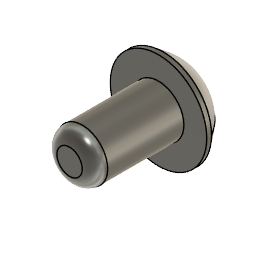
Assembled Parallel Gripper (Autodesk Fusion 360 archive; units mm, degrees)
design "P.Gripper_Pin"
part number: 2026-07-30-16-02-04-406
Autodesk Fusion 360 part; units mm, degrees
sketch "Sketch2" plane through (0, 0, 0) normal (0, 0, 1) x (1, 0, 0)
  line L0 (0, 20) -> (3.8, 20)
  line L1 (3.8, 20) -> (3.8, 20.38)
  spline S0 degree 5 poles (3.8, 20.38) (3.7593, 20.4429) (3.678, 20.5664) (3.5568, 20.7451) (3.3966, 20.9696) (3.1989, 21.2259) (3.0039, 21.4555) (2.812, 21.6558) (2.6234, 21.8246) (2.438, 21.9621) (2.2557, 22.0702) (2.1121, 22.1349) (2.0056, 22.1719) (1.9351, 22.1915) (1.9, 22.2) knots 0 0 0 0 0 0 0.1 0.2 0.3 0.4 0.5 0.6 0.7 0.8 0.9 1 1 1 1 1 1
  line L2 (0, 20) -> (0, 22.2)
  line L3 (0, 22.2) -> (1.9, 22.2)
  point P0 (2.7411, 21.7155)
  dimension "d4" = 3.8
  dimension "d5" = 0.38
  dimension "d6" = 2.2
  dimension "d7" = 1.9
  constraint horizontal L0
  constraint perpendicular L0 L1
  constraint perpendicular L0 L2
  constraint perpendicular L2 L3
  measures "d4" distance of L0.start L0.end
  measures "d5" distance of L0.end L1.end
  measures "d6" distance of L0.start L2.end
  measures "d7" distance of L2.end S0.end
revolve "Revolve1" add sketch "Sketch2" angle 360 about axis through (0, 20, 0) along (0, 1, 0)
sketch "Sketch3" plane through (0, 22.2, 0) normal (0, 1, 0) x (-1, 0, 0)
  circle A0 centre (0, 0) radius 1.9
  line L0 (0.7217, -1.25) -> (1.4434, 0)
  line L1 (1.4434, 0) -> (0.7217, 1.25)
  line L2 (0.7217, 1.25) -> (-0.7217, 1.25)
  line L3 (-0.7217, 1.25) -> (-1.4434, 0)
  line L4 (-1.4434, 0) -> (-0.7217, -1.25)
  line L5 (-0.7217, -1.25) -> (0.7217, -1.25)
  dimension "d9" = 2.5
  constraint coincident A0.centre origin
  measures "d9" distance of L0.start L1.end
extrude "Extrude2" cut sketch "Sketch3" against normal blind 2 contours L0 L1 L2 L3 L4 L5
sketch "Sketch4" plane through (0, 20, 0) normal (0, -1, 0) x (1, 0, 0)
  circle A0 centre (0, 0) radius 3.8
  circle A1 centre (0, 0) radius 2
  dimension "d14" = 4
  constraint coincident A0.centre A1.centre
  measures "d14" diameter of A1
extrude "Extrude3" add sketch "Sketch4" along normal blind 7 contours A1
fillet "Fillet2" radius 1 1 edges at (-1.8647, 13, -0.7232)

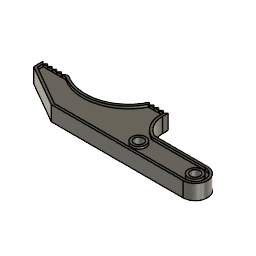
design "P.Gripper_gripper"
part number: 2026-07-22-21-10-46-323
Autodesk Fusion 360 part; units mm, degrees
sketch "Sketch1" plane through (0, 0, 0) normal (0, 0, 1) x (1, 0, 0)
  line L0 (35, 0) -> (-35, 0)
  line L1 (-35, 0) -> (-57.0836, 12.75)
  line L2 (-35, 0) -> (-60.5, 0) construction
  line L3 (-57.0836, 12.75) -> (-57.0836, 17.75)
  line L4 (-57.0836, 17.75) -> (-43.4836, 17.75)
  line L5 (-10, 27.12) -> (0.01, 27.12)
  arc A0 (-43.4836, 17.75) -> (-10, 27.12) centre (-30.7999, 36.9365) ccw
  line L6 (35, 0) -> (35, 13)
  arc A1 (35, 0) -> (35, 13) centre (35, 6.5) ccw
  line L7 (35, 13) -> (6.8247, 13)
  line L8 (0.01, 27.12) -> (0.01, 24.12)
  arc A2 (0.01, 24.12) -> (6.8247, 13) centre (12.49, 24.12) ccw
  dimension "d1" = 70
  dimension "d2" = 30
  dimension "d3" = 25.5
  dimension "d4" = 5
  dimension "d5" = 13.6
  dimension "d6" = 10.01
  dimension "d7" = 27.12
  dimension "d8" = 23
  dimension "d9" = 13
  dimension "d10" = 3
  constraint midpoint L0 origin
  constraint horizontal L0
  constraint horizontal L2
  constraint vertical L3
  constraint perpendicular L3 L4
  constraint horizontal L5
  constraint perpendicular L0 L6
  constraint midpoint L6 A1.centre
  constraint tangent A1 L7
  constraint perpendicular L5 L8
  constraint tangent L8 A2
  measures "d1" distance of L0.start L0.end
  measures "d2" angle of L1 L2
  measures "d3" distance of L0.end L1.end
  measures "d4" distance of L1.end L3.end
  measures "d5" distance of L3.end L4.end
  measures "d6" distance of L5.start L5.end
  measures "d7" distance of L0 L5
  measures "d8" radius of A0
  measures "d9" distance of L0.start L6.end
  measures "d10" distance of L5.end L8.end
extrude "Extrude1" add sketch "Sketch1" along normal mid plane 8
fillet "Fillet1" radius 2 1 edges at (6.8247, 13, 0)
sketch "Sketch2" plane through (0, 0, 4) normal (0, 0, 1) x (-1, 0, 0)
  arc A0 (-35, 0) -> (-35, -13) centre (-35, -6.5) ccw
  line L0 (-35, -13) -> (-7.3271, -13)
  arc A1 (-6.3418, -13.2595) -> (-7.3271, -13) centre (-7.3271, -15) ccw
  arc A2 (-0.01, -24.12) -> (-6.3418, -13.2595) centre (-12.49, -24.12) ccw
  line L1 (-0.01, -24.12) -> (-0.01, -27.12)
  line L2 (-0.01, -27.12) -> (10, -27.12)
  arc A3 (43.4836, -17.75) -> (10, -27.12) centre (30.7999, -36.9365) ccw
  line L3 (43.4836, -17.75) -> (57.0836, -17.75)
  line L4 (57.0836, -17.75) -> (57.0836, -12.75)
  line L5 (57.0836, -12.75) -> (35, 0)
  line L6 (35, 0) -> (-35, 0)
  circle A4 centre (-35, -6.5) radius 2.5
  line L7 (-35, -6.5) -> (-5, -6.5)
  circle A5 centre (-5, -6.5) radius 2.5
  dimension "d15" = 5
  dimension "d16" = 30
  dimension "d17" = 5
  constraint concentric A0 A4
  constraint coincident A0.centre A4.centre
  constraint parallel L0 L7
  constraint coincident L7.end A5.centre
  measures "d15" diameter of A4
  measures "d16" distance of A0.centre L7.end
  measures "d17" diameter of A5
extrude "Extrude2" cut sketch "Sketch2" against normal blind 16 contours A4 | A5
sketch "Sketch3" plane through (0, 0, 4) normal (0, 0, 1) x (-1, 0, 0)
  circle A0 centre (-5, -6.5) radius 2.5
  circle A1 centre (-35, -6.5) radius 2.5
  arc A2 (-35, 0) -> (-35, -13) centre (-35, -6.5) ccw
  line L0 (-35, -13) -> (-7.3271, -13)
  arc A3 (-6.3418, -13.2595) -> (-7.3271, -13) centre (-7.3271, -15) ccw
  arc A4 (-0.01, -24.12) -> (-6.3418, -13.2595) centre (-12.49, -24.12) ccw
  line L1 (-0.01, -24.12) -> (-0.01, -27.12)
  line L2 (-0.01, -27.12) -> (10, -27.12)
  arc A5 (43.4836, -17.75) -> (10, -27.12) centre (30.7999, -36.9365) ccw
  line L3 (43.4836, -17.75) -> (57.0836, -17.75)
  line L4 (57.0836, -17.75) -> (57.0836, -12.75)
  line L5 (57.0836, -12.75) -> (35, 0)
  line L6 (35, 0) -> (-35, 0)
  arc A6 (43.8541, -16.5) -> (9.2223, -25.87) centre (30.7999, -36.9365) ccw
  line L7 (1.24, -25.87) -> (9.2223, -25.87)
  line L8 (1.24, -24.12) -> (1.24, -25.87)
  arc A7 (1.24, -24.12) -> (-5.726, -12.1718) centre (-12.49, -24.12) ccw
  arc A8 (-5.726, -12.1718) -> (-7.3271, -11.75) centre (-7.3271, -15) ccw
  line L9 (-35, -11.75) -> (-7.3271, -11.75)
  arc A9 (-35, -1.25) -> (-35, -11.75) centre (-35, -6.5) ccw
  line L10 (34.6651, -1.25) -> (-35, -1.25)
  line L11 (55.8336, -13.4717) -> (34.6651, -1.25)
  line L12 (55.8336, -16.5) -> (55.8336, -13.4717)
  line L13 (43.8541, -16.5) -> (55.8336, -16.5)
  dimension "d21" = -1.25
extrude "Extrude3" cut sketch "Sketch3" against normal blind 1.25 contours A6 L7 L8 A7 A8 L9 A9 L10 L11 L12 L13
sketch "Sketch4" plane through (0, 0, 2.75) normal (0, 0, 1) x (-1, 0, 0)
  circle A0 centre (-35, -6.5) radius 2.5
  circle A1 centre (-5, -6.5) radius 2.5
  line L0 (1.24, -24.12) -> (1.24, -25.87)
  line L1 (1.24, -25.87) -> (9.2223, -25.87)
  arc A2 (43.8541, -16.5) -> (9.2223, -25.87) centre (30.7999, -36.9365) ccw
  line L2 (43.8541, -16.5) -> (55.8336, -16.5)
  line L3 (55.8336, -16.5) -> (55.8336, -13.4717)
  line L4 (55.8336, -13.4717) -> (34.6651, -1.25)
  line L5 (34.6651, -1.25) -> (-35, -1.25)
  arc A3 (-35, -1.25) -> (-35, -11.75) centre (-35, -6.5) ccw
  line L6 (-35, -11.75) -> (-7.3271, -11.75)
  arc A4 (-5.726, -12.1718) -> (-7.3271, -11.75) centre (-7.3271, -15) ccw
  arc A5 (1.24, -24.12) -> (-5.726, -12.1718) centre (-12.49, -24.12) ccw
  circle A6 centre (-5, -6.5) radius 3.75
  circle A7 centre (-35, -6.5) radius 3.75
  dimension "d24" = 1.25
  dimension "d25" = 1.25
extrude "Extrude4" add sketch "Sketch4" along normal blind 1.25 contours A6 | A7
sketch "Sketch5" plane through (0, 0, -4) normal (0, 0, -1) x (1, 0, 0)
  circle A0 centre (5, -6.5) radius 2.5
  circle A1 centre (35, -6.5) radius 2.5
  arc A2 (35, -13) -> (35, 0) centre (35, -6.5) ccw
  line L0 (35, 0) -> (-35, 0)
  line L1 (-35, 0) -> (-57.0836, -12.75)
  line L2 (-57.0836, -12.75) -> (-57.0836, -17.75)
  line L3 (-57.0836, -17.75) -> (-43.4836, -17.75)
  arc A3 (-10, -27.12) -> (-43.4836, -17.75) centre (-30.7999, -36.9365) ccw
  line L4 (-10, -27.12) -> (0.01, -27.12)
  line L5 (0.01, -27.12) -> (0.01, -24.12)
  arc A4 (6.3418, -13.2595) -> (0.01, -24.12) centre (12.49, -24.12) ccw
  arc A5 (7.3271, -13) -> (6.3418, -13.2595) centre (7.3271, -15) ccw
  line L6 (7.3271, -13) -> (35, -13)
  circle A6 centre (5, -6.5) radius 3.75
  circle A7 centre (35, -6.5) radius 3.75
  line L7 (-55.8336, -16.5) -> (-43.8541, -16.5)
  arc A8 (-9.2223, -25.87) -> (-43.8541, -16.5) centre (-30.7999, -36.9365) ccw
  line L8 (-9.2223, -25.87) -> (-1.24, -25.87)
  line L9 (-1.24, -25.87) -> (-1.24, -24.12)
  arc A9 (5.726, -12.1718) -> (-1.24, -24.12) centre (12.49, -24.12) ccw
  arc A10 (7.3271, -11.75) -> (5.726, -12.1718) centre (7.3271, -15) ccw
  line L10 (7.3271, -11.75) -> (35, -11.75)
  arc A11 (35, -11.75) -> (35, -1.25) centre (35, -6.5) ccw
  line L11 (35, -1.25) -> (-34.6651, -1.25)
  line L12 (-34.6651, -1.25) -> (-55.8336, -13.4717)
  line L13 (-55.8336, -13.4717) -> (-55.8336, -16.5)
  dimension "d28" = 1.25
  dimension "d29" = 1.25
  dimension "d30" = 1.25
extrude "Extrude5" cut sketch "Sketch5" against normal blind 1.25 contours L7 A8 L8 L9 A9 A10 L10 A11 L11 L12 L13
sketch "Sketch7" plane through (0, 0, 4) normal (0, 0, 1) x (-1, 0, 0)
  line L0 (9.2223, -25.87) -> (1.24, -25.87)
  line L1 (1.24, -25.87) -> (1.24, -24.12)
  arc A0 (1.24, -24.12) -> (-5.726, -12.1718) centre (-12.49, -24.12) ccw
  arc A1 (-5.726, -12.1718) -> (-7.3271, -11.75) centre (-7.3271, -15) ccw
  line L2 (-7.3271, -11.75) -> (-35, -11.75)
  arc A2 (-35, -1.25) -> (-35, -11.75) centre (-35, -6.5) ccw
  line L3 (-35, -1.25) -> (34.6651, -1.25)
  line L4 (34.6651, -1.25) -> (55.8336, -13.4717)
  line L5 (55.8336, -13.4717) -> (55.8336, -16.5)
  line L6 (55.8336, -16.5) -> (43.8541, -16.5)
  arc A3 (43.8541, -16.5) -> (9.2223, -25.87) centre (30.7999, -36.9365) ccw
  arc A4 (-35, 0) -> (-35, -13) centre (-35, -6.5) ccw
  line L7 (-35, -13) -> (-7.3271, -13)
  arc A5 (-6.3418, -13.2595) -> (-7.3271, -13) centre (-7.3271, -15) ccw
  arc A6 (-0.01, -24.12) -> (-6.3418, -13.2595) centre (-12.49, -24.12) ccw
  line L8 (-0.01, -24.12) -> (-0.01, -27.12)
  line L9 (-0.01, -27.12) -> (10, -27.12)
  arc A7 (43.4836, -17.75) -> (10, -27.12) centre (30.7999, -36.9365) ccw
  line L10 (43.4836, -17.75) -> (57.0836, -17.75)
  line L11 (57.0836, -17.75) -> (57.0836, -12.75)
  line L12 (57.0836, -12.75) -> (35, 0)
  line L13 (35, 0) -> (-35, 0)
  line L14 (42, -16.7) -> (58, -16.7)
  line L15 (57.0836, -17.75) -> (55.8816, -16.5479)
  line L16 (57.0836, -17.75) -> (58.7836, -17.75) construction
  line L17 (55.8816, -16.5479) -> (54.6795, -17.75)
  line L18 (54.6795, -17.75) -> (53.4525, -16.523)
  line L19 (53.4525, -16.523) -> (52.2254, -17.75)
  line L20 (52.2254, -17.75) -> (50.9984, -16.523)
  line L21 (50.9984, -16.523) -> (49.7714, -17.75)
  line L22 (49.7714, -17.75) -> (48.5214, -16.5)
  line L23 (48.5214, -16.5) -> (47.2714, -17.75)
  line L24 (47.2714, -17.75) -> (46.0214, -16.5)
  line L25 (46.0214, -16.5) -> (44.7714, -17.75)
  line L26 (44.7714, -17.75) -> (43.5093, -16.4879)
  point P0 (50, -16.7)
  dimension "d33" = 0.2
  dimension "d34" = 135
  dimension "d35" = 1.7
  dimension "d37" = 90
  constraint midpoint L14 P0
  constraint perpendicular L11 L14
  constraint horizontal L16
  constraint coincident L10.end L11.start
  constraint coincident L10 L17.end
  constraint perpendicular L15 L17
  constraint coincident L10 L19.end
  constraint perpendicular L18 L19
  constraint coincident L10 L21.end
  constraint perpendicular L20 L21
  constraint coincident L6 L22.end
  constraint perpendicular L21 L22
  constraint coincident L10 L23.end
  constraint perpendicular L22 L23
  constraint coincident L6 L24.end
  constraint perpendicular L23 L24
  constraint coincident L10 L25.end
  constraint perpendicular L24 L25
  measures "d33" distance of L6 L14
  measures "d34" angle of L15 L16
  measures "d35" distance of L10.end L15.end
  measures "d37" angle of L25 L26
extrude "Extrude6" cut sketch "Sketch7" against normal blind 16 contours L10 L14 L24 L25 | L10 L14 L22 L23 | L10 L14 L20 L21 | L10 L14 L18 L19 | L10 L14 L15 L17
sketch "Sketch8" plane through (0, 0, 4) normal (0, 0, 1) x (-1, 0, 0)
  line L0 (9.2223, -25.87) -> (1.24, -25.87)
  line L1 (1.24, -25.87) -> (1.24, -24.12)
  arc A0 (1.24, -24.12) -> (-5.726, -12.1718) centre (-12.49, -24.12) ccw
  arc A1 (-5.726, -12.1718) -> (-7.3271, -11.75) centre (-7.3271, -15) ccw
  line L2 (-7.3271, -11.75) -> (-35, -11.75)
  arc A2 (-35, -1.25) -> (-35, -11.75) centre (-35, -6.5) ccw
  line L3 (-35, -1.25) -> (34.6651, -1.25)
  line L4 (34.6651, -1.25) -> (55.8336, -13.4717)
  line L5 (55.8336, -13.4717) -> (55.8336, -16.5)
  line L6 (55.8336, -16.5) -> (43.8541, -16.5)
  arc A3 (43.8541, -16.5) -> (9.2223, -25.87) centre (30.7999, -36.9365) ccw
  line L7 (44.7714, -17.75) -> (45.8214, -16.7)
  line L8 (45.8214, -16.7) -> (46.2214, -16.7)
  line L9 (46.2214, -16.7) -> (47.2714, -17.75)
  line L10 (47.2714, -17.75) -> (48.3214, -16.7)
  line L11 (48.3214, -16.7) -> (48.7214, -16.7)
  line L12 (48.7214, -16.7) -> (49.7714, -17.75)
  line L13 (49.7714, -17.75) -> (50.8214, -16.7)
  line L14 (50.8214, -16.7) -> (51.1754, -16.7)
  line L15 (51.1754, -16.7) -> (52.2254, -17.75)
  line L16 (52.2254, -17.75) -> (53.2754, -16.7)
  line L17 (53.2754, -16.7) -> (53.6295, -16.7)
  line L18 (53.6295, -16.7) -> (54.6795, -17.75)
  line L19 (54.6795, -17.75) -> (55.7295, -16.7)
  line L20 (55.7295, -16.7) -> (56.0336, -16.7)
  line L21 (56.0336, -16.7) -> (57.0836, -17.75)
  line L22 (57.0836, -17.75) -> (57.0836, -12.75)
  line L23 (57.0836, -12.75) -> (35, 0)
  line L24 (35, 0) -> (-35, 0)
  arc A4 (-35, 0) -> (-35, -13) centre (-35, -6.5) ccw
  line L25 (-35, -13) -> (-7.3271, -13)
  arc A5 (-6.3418, -13.2595) -> (-7.3271, -13) centre (-7.3271, -15) ccw
  arc A6 (-0.01, -24.12) -> (-6.3418, -13.2595) centre (-12.49, -24.12) ccw
  line L26 (-0.01, -24.12) -> (-0.01, -27.12)
  line L27 (-0.01, -27.12) -> (10, -27.12)
  arc A7 (43.4836, -17.75) -> (10, -27.12) centre (30.7999, -36.9365) ccw
  line L28 (43.4836, -17.75) -> (44.7714, -17.75)
  line L29 (-1.01, -26.07) -> (11, -26.07)
  line L30 (10, -27.12) -> (8.75, -25.87)
  line L31 (10, -27.12) -> (11.7678, -27.12) construction
  line L32 (8.75, -25.87) -> (7.5, -27.12)
  line L33 (7.5, -27.12) -> (6.25, -25.87)
  line L34 (6.25, -25.87) -> (4.995, -27.125)
  line L35 (4.995, -27.125) -> (3.74, -25.87)
  line L36 (3.74, -25.87) -> (2.49, -27.12)
  line L37 (2.49, -27.12) -> (1.24, -25.87)
  line L38 (1.24, -25.87) -> (-0.01, -27.12)
  point P0 (4.995, -26.07)
  dimension "d40" = 0.2
  dimension "d41" = 135
  constraint midpoint L29 P0
  constraint parallel L27 L29
  constraint horizontal L31
  constraint coincident L27.end A7.end
  constraint coincident L0 L30.end
  constraint coincident L27 L32.end
  constraint perpendicular L30 L32
  constraint perpendicular L32 L33
  constraint perpendicular L33 L34
  constraint coincident L0 L35.end
  constraint perpendicular L34 L35
  constraint coincident L27 L36.end
  constraint perpendicular L35 L36
  constraint coincident L0.end L1.start
  constraint perpendicular L36 L37
  constraint coincident L26.end L27.start
  measures "d40" distance of L0 L29
  measures "d41" angle of L30 L31
extrude "Extrude7" cut sketch "Sketch8" against normal blind 16 contours L27 L29 L30 L32 | L27 L29 L33 L34 | L27 L29 L35 L36 | L27 L29 L37 L38

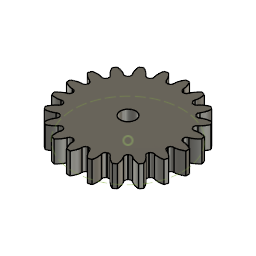
design "Spur Gear 20 teeth"
description: Spur Gear; Module: 1.75; Num Teeth: 20; Pressure Angle: 20.0; Backlash: 0.00 mm
part number: 2026-07-22-22-21-55-407
Autodesk Fusion 360 part; units mm, degrees
sketch "Base Circle" plane through (0, 0, 0) normal (0, 0, 1) x (1, 0, 0)
  circle A0 centre (0, 0) radius 15.4753
  circle A1 centre (0, 0) radius 2.5
extrude "Extrude1" add sketch "Base Circle" along normal blind 7
sketch "Gear Tooth" plane through (0, 0, 0) normal (0, 0, 1) x (1, 0, 0)
  spline S0 degree 5 poles (16.3729, -1.5344) (16.3811, -1.5352) (16.3975, -1.5365) (16.4221, -1.5378) (16.455, -1.5384) (16.4962, -1.5373) (16.5375, -1.535) (16.5788, -1.532) (16.6201, -1.5285) (16.6614, -1.5248) (16.7028, -1.5207) (16.7442, -1.5163) (16.7855, -1.5114) (16.8269, -1.5059) (16.8683, -1.4998) (16.9098, -1.4931) (16.9512, -1.486) (16.9926, -1.4784) (17.034, -1.4706) (17.0754, -1.4623) (17.1168, -1.4538) (17.1582, -1.4449) (17.1996, -1.4356) (17.241, -1.426) (17.2824, -1.416) (17.3238, -1.4057) (17.3651, -1.395) (17.4065, -1.3839) (17.4478, -1.3726) (17.4891, -1.361) (17.5304, -1.349) (17.5717, -1.3368) (17.613, -1.3243) (17.6542, -1.3114) (17.6955, -1.2983) (17.7367, -1.2849) (17.7779, -1.2711) (17.8191, -1.2571) (17.8602, -1.2429) (17.9013, -1.2283) (17.9424, -1.2135) (17.9835, -1.1984) (18.0246, -1.183) (18.0656, -1.1674) (18.1066, -1.1515) (18.1475, -1.1354) (18.1885, -1.119) (18.2294, -1.1023) (18.2703, -1.0854) (18.3111, -1.0682) (18.3519, -1.0508) (18.3927, -1.0331) (18.4334, -1.0152) (18.4742, -0.9971) (18.5148, -0.9787) (18.5555, -0.96) (18.5961, -0.9412) (18.6367, -0.922) (18.6772, -0.9027) (18.7177, -0.8831) (18.7582, -0.8633) (18.7986, -0.8433) (18.839, -0.823) (18.8793, -0.8025) (18.9196, -0.7818) (18.9598, -0.7608) (19.0001, -0.7396) (19.0402, -0.7182) (19.0804, -0.6966) (19.1204, -0.6748) (19.1605, -0.6527) (19.1925, -0.6349) (19.2164, -0.6215) (19.2324, -0.6124) (19.2404, -0.6079) knots 0 0 0 0 0 0 0.01428571 0.02857143 0.04285714 0.05714286 0.07142857 0.08571429 0.1 0.11428571 0.12857143 0.14285714 0.15714286 0.17142857 0.18571429 0.2 0.21428571 0.22857143 0.24285714 0.25714286 0.27142857 0.28571429 0.3 0.31428571 0.32857143 0.34285714 0.35714286 0.37142857 0.38571429 0.4 0.41428571 0.42857143 0.44285714 0.45714286 0.47142857 0.48571429 0.5 0.51428571 0.52857143 0.54285714 0.55714286 0.57142857 0.58571429 0.6 0.61428571 0.62857143 0.64285714 0.65714286 0.67142857 0.68571429 0.7 0.71428571 0.72857143 0.74285714 0.75714286 0.77142857 0.78571429 0.8 0.81428571 0.82857143 0.84285714 0.85714286 0.87142857 0.88571429 0.9 0.91428571 0.92857143 0.94285714 0.95714286 0.97142857 0.98571429 1 1 1 1 1 1
  spline S1 degree 5 poles (16.3729, 1.5344) (16.3811, 1.5352) (16.3975, 1.5365) (16.4221, 1.5378) (16.455, 1.5384) (16.4962, 1.5373) (16.5375, 1.535) (16.5788, 1.532) (16.6201, 1.5285) (16.6614, 1.5248) (16.7028, 1.5207) (16.7442, 1.5163) (16.7855, 1.5114) (16.8269, 1.5059) (16.8683, 1.4998) (16.9098, 1.4931) (16.9512, 1.486) (16.9926, 1.4784) (17.034, 1.4706) (17.0754, 1.4623) (17.1168, 1.4538) (17.1582, 1.4449) (17.1996, 1.4356) (17.241, 1.426) (17.2824, 1.416) (17.3238, 1.4057) (17.3651, 1.395) (17.4065, 1.3839) (17.4478, 1.3726) (17.4891, 1.361) (17.5304, 1.349) (17.5717, 1.3368) (17.613, 1.3243) (17.6542, 1.3114) (17.6955, 1.2983) (17.7367, 1.2849) (17.7779, 1.2711) (17.8191, 1.2571) (17.8602, 1.2429) (17.9013, 1.2283) (17.9424, 1.2135) (17.9835, 1.1984) (18.0246, 1.183) (18.0656, 1.1674) (18.1066, 1.1515) (18.1475, 1.1354) (18.1885, 1.119) (18.2294, 1.1023) (18.2703, 1.0854) (18.3111, 1.0682) (18.3519, 1.0508) (18.3927, 1.0331) (18.4334, 1.0152) (18.4742, 0.9971) (18.5148, 0.9787) (18.5555, 0.96) (18.5961, 0.9412) (18.6367, 0.922) (18.6772, 0.9027) (18.7177, 0.8831) (18.7582, 0.8633) (18.7986, 0.8433) (18.839, 0.823) (18.8793, 0.8025) (18.9196, 0.7818) (18.9598, 0.7608) (19.0001, 0.7396) (19.0402, 0.7182) (19.0804, 0.6966) (19.1204, 0.6748) (19.1605, 0.6527) (19.1925, 0.6349) (19.2164, 0.6215) (19.2324, 0.6124) (19.2404, 0.6079) knots 0 0 0 0 0 0 0.01428571 0.02857143 0.04285714 0.05714286 0.07142857 0.08571429 0.1 0.11428571 0.12857143 0.14285714 0.15714286 0.17142857 0.18571429 0.2 0.21428571 0.22857143 0.24285714 0.25714286 0.27142857 0.28571429 0.3 0.31428571 0.32857143 0.34285714 0.35714286 0.37142857 0.38571429 0.4 0.41428571 0.42857143 0.44285714 0.45714286 0.47142857 0.48571429 0.5 0.51428571 0.52857143 0.54285714 0.55714286 0.57142857 0.58571429 0.6 0.61428571 0.62857143 0.64285714 0.65714286 0.67142857 0.68571429 0.7 0.71428571 0.72857143 0.74285714 0.75714286 0.77142857 0.78571429 0.8 0.81428571 0.82857143 0.84285714 0.85714286 0.87142857 0.88571429 0.9 0.91428571 0.92857143 0.94285714 0.95714286 0.97142857 0.98571429 1 1 1 1 1 1
  arc A0 (19.2404, -0.6079) -> (19.2404, 0.6079) centre (0, 0) ccw
  line L0 (15.3978, -1.443) -> (16.3729, -1.5344)
  line L1 (15.3978, 1.443) -> (16.3729, 1.5344)
  line L2 (15.3978, -1.443) -> (15.3978, 1.443)
  point P0 (16.5743, -1.5322)
  point P1 (16.7774, -1.5123)
  point P2 (16.9814, -1.4804)
  point P3 (17.1861, -1.4386)
  point P4 (17.3912, -1.388)
  point P5 (17.5968, -1.3291)
  point P6 (17.8026, -1.2627)
  point P7 (18.0085, -1.189)
  point P8 (18.2144, -1.1084)
  point P9 (18.4202, -1.021)
  point P10 (18.6258, -0.9271)
  point P11 (18.8311, -0.8269)
  point P12 (19.036, -0.7205)
  point P13 (16.5743, 1.5322)
  point P14 (16.7774, 1.5123)
  point P15 (16.9814, 1.4804)
  point P16 (17.1861, 1.4386)
  point P17 (17.3912, 1.388)
  point P18 (17.5968, 1.3291)
  point P19 (17.8026, 1.2627)
  point P20 (18.0085, 1.189)
  point P21 (18.2144, 1.1084)
  point P22 (18.4202, 1.021)
  point P23 (18.6258, 0.9271)
  point P24 (18.8311, 0.8269)
  point P25 (19.036, 0.7205)
extrude "Extrude2" add sketch "Gear Tooth" along normal blind 7
fillet "Fillet1" radius 1 2 edges at (15.4077, -1.444, 3.5) (15.4077, 1.444, 3.5)
pattern_circular "C-Pattern1" count 20 over 360 about axis through (0, 0, 0) along (0, 0, 1) of "Extrude2", "Fillet1"
sketch "Diametrial Pitch Circle" plane through (0, 0, 0) normal (0, 0, 1) x (1, 0, 0)
  circle A0 centre (0, 0) radius 17.5 construction

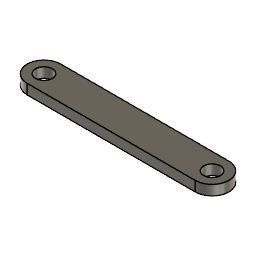
design "P.Gripper_Clamp"
part number: 2026-07-22-21-07-09-369
Autodesk Fusion 360 part; units mm, degrees
sketch "Sketch1" plane through (0, 0, 0) normal (0, 0, 1) x (1, 0, 0)
  line L0 (-25, -5) -> (25, -5)
  arc A0 (25, -5) -> (25, 5) centre (25, 0) ccw
  line L1 (25, 5) -> (-25, 5)
  arc A1 (-25, 5) -> (-25, -5) centre (-25, 0) ccw
  line L2 (-25, 0) -> (25, 0) construction
  dimension "d1" = 50
  dimension "d2" = 5
  constraint tangent L0 A0
  constraint tangent A0 L1
  constraint parallel L0 L1
  constraint tangent L1 A1
  constraint tangent L0 A1
  constraint horizontal L2
  constraint midpoint L2 origin
  measures "d1" distance of A1.centre A0.centre
  measures "d2" radius of A1
extrude "Extrude1" add sketch "Sketch1" along normal blind 3
sketch "Sketch2" plane through (0, 0, 3) normal (0, 0, 1) x (-1, 0, 0)
  arc A0 (25, -5) -> (25, 5) centre (25, 0) ccw
  line L0 (25, 5) -> (-25, 5)
  arc A1 (-25, 5) -> (-25, -5) centre (-25, 0) ccw
  line L1 (-25, -5) -> (25, -5)
  circle A2 centre (25, 0) radius 2.5
  circle A3 centre (-25, 0) radius 2.5
  dimension "d5" = 5
  dimension "d6" = 5
  constraint concentric A0 A2
  constraint concentric A1 A3
  measures "d5" diameter of A2
  measures "d6" diameter of A3
extrude "Extrude2" cut sketch "Sketch2" against normal blind 3 contours A2 | A3

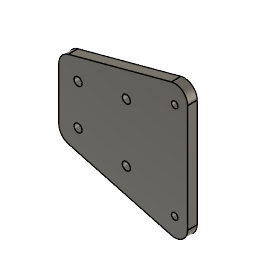
design "Parallel Gripper"
part number: 2026-07-22-20-24-16-887
Autodesk Fusion 360 part; units mm, degrees
sketch "Sketch1" plane through (0, 0, 0) normal (0, 1, 0) x (1, 0, 0)
  line L0 (-80, 0) -> (-80, -16.3617)
  line L1 (-74.0709, -24.089) -> (-10.0709, -41.241)
  line L2 (0, -33.5137) -> (0, 0)
  line L3 (0, 0) -> (-80, 0)
  arc A0 (-80, -16.3617) -> (-74.0709, -24.089) centre (-72, -16.3617) ccw
  arc A1 (-10.0709, -41.241) -> (0, -33.5137) centre (-8, -33.5137) ccw
  point P0 (-80, -22.5)
  point P1 (0, -43.94)
  dimension "d1" = 22.5
  dimension "d2" = 43.94
  dimension "d3" = 80
  dimension "d4" = 8
  dimension "d5" = 8
  constraint vertical L0
  constraint parallel L0 L2
  constraint coincident L2.end L3.start
  constraint perpendicular L0 L3
  constraint coincident P0 L0
  constraint coincident P0 L1
  constraint tangent L0 A0
  constraint tangent L1 A0
  constraint coincident P1 L1
  constraint coincident P1 L2
  constraint tangent L1 A1
  constraint tangent L2 A1
  measures "d1" distance of L0.start P0
  measures "d2" distance of P1 L2.end
  measures "d3" distance of L0.start L2.end
  measures "d4" radius of A0
  measures "d5" radius of A1
extrude "Extrude1" add sketch "Sketch1" along normal mid plane 6
mirror "Mirror1" about plane through (0, 0, 0) normal (0, 0, 1) of bodies 1 merged
sketch "Sketch2" plane through (0, -3, 0) normal (0, -1, 0) x (1, 0, 0)
  arc A0 (0, 33.5137) -> (-10.0709, 41.241) centre (-8, 33.5137) ccw
  line L0 (-10.0709, 41.241) -> (-74.0709, 24.089)
  arc A1 (-74.0709, 24.089) -> (-80, 16.3617) centre (-72, 16.3617) ccw
  line L1 (-80, 16.3617) -> (-80, -16.3617)
  arc A2 (-80, -16.3617) -> (-74.0709, -24.089) centre (-72, -16.3617) ccw
  line L2 (-74.0709, -24.089) -> (-10.0709, -41.241)
  arc A3 (-10.0709, -41.241) -> (0, -33.5137) centre (-8, -33.5137) ccw
  line L3 (0, -33.5137) -> (0, 33.5137)
  line L4 (-160, 0) -> (0, 0)
  circle A4 centre (-8, 30) radius 2
  circle A5 centre (-38, 18) radius 2.5
  circle A6 centre (-68, 12.5) radius 2.5
  circle A7 centre (-68, -12.5) radius 2.5
  circle A8 centre (-38, -18) radius 2.5
  circle A9 centre (-8, -30) radius 2
  point P0 (-80, 0)
  dimension "d12" = 4
  dimension "d13" = 5
  dimension "d14" = 5
  dimension "d15" = 12
  dimension "d16" = 12.5
  dimension "d17" = 18
  dimension "d18" = 30
  dimension "d19" = 8
  dimension "d20" = 38
  constraint midpoint L4 P0
  constraint coincident L1 P0
  constraint coincident L4.end origin
  constraint perpendicular L3 L4
  constraint symmetric L4 A4 A9
  constraint symmetric L4 A5 A8
  constraint symmetric L4 A6 A7
  measures "d12" diameter of A4
  measures "d13" diameter of A5
  measures "d14" diameter of A6
  measures "d15" distance of L1 A6.centre
  measures "d16" distance of L4 A6.centre
  measures "d17" distance of L4 A5.centre
  measures "d18" distance of L4 A4.centre
  measures "d19" distance of L3 A4.centre
  measures "d20" distance of L3 A8.centre
extrude "Extrude2" cut sketch "Sketch2" against normal blind 6 contours A4 | A5 | A6 | A7 | A8 | A9

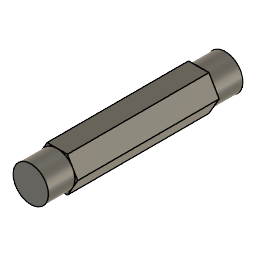
design "Parallel Gripper_Aligner"
part number: 2026-07-22-21-01-51-202
Autodesk Fusion 360 part; units mm, degrees
sketch "Sketch1" plane through (0, 0, 0) normal (0, 1, 0) x (1, 0, 0)
  line L0 (-1.1547, 2) -> (-2.3094, 0)
  line L1 (-2.3094, 0) -> (-1.1547, -2)
  line L2 (-1.1547, -2) -> (1.1547, -2)
  line L3 (1.1547, -2) -> (2.3094, 0)
  line L4 (2.3094, 0) -> (1.1547, 2)
  line L5 (1.1547, 2) -> (-1.1547, 2)
  dimension "d1" = 4
  measures "d1" distance of L2 L5
extrude "Extrude1" add sketch "Sketch1" along normal blind 16
sketch "Sketch2" plane through (0, 0, 0) normal (0, -1, 0) x (1, 0, 0)
  line L0 (-1.1547, -2) -> (1.1547, -2)
  line L1 (1.1547, -2) -> (2.3094, 0)
  line L2 (2.3094, 0) -> (1.1547, 2)
  line L3 (1.1547, 2) -> (-1.1547, 2)
  line L4 (-1.1547, 2) -> (-2.3094, 0)
  line L5 (-2.3094, 0) -> (-1.1547, -2)
  circle A0 centre (0, 0) radius 2
  constraint coincident A0.centre origin
extrude "Extrude2" add sketch "Sketch2" along normal blind 3 contours A0
sketch "Sketch3" plane through (0, 16, 0) normal (0, 1, 0) x (-1, 0, 0)
  line L0 (-1.1547, -2) -> (1.1547, -2)
  line L1 (1.1547, -2) -> (2.3094, 0)
  line L2 (2.3094, 0) -> (1.1547, 2)
  line L3 (1.1547, 2) -> (-1.1547, 2)
  line L4 (-1.1547, 2) -> (-2.3094, 0)
  line L5 (-2.3094, 0) -> (-1.1547, -2)
  circle A0 centre (0, 0) radius 2
  constraint coincident A0.centre origin
  constraint tangent L0 A0
extrude "Extrude3" add sketch "Sketch3" along normal blind 3 contours A0
